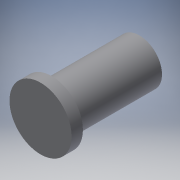
# Autodesk Inventor part: PinLarge
Saved by Autodesk Inventor 2016 (Build 200138000, 138)
## iProperties
Created: 2017-02-20
Part Number: PinLarge
Material: Generic
Document SubType Name: Modeling
Designer: Owner
Density: 1 g/cm^3
Appearance: Default
Author: Owner
Autodesk Inventor part; units mm, degrees
ref_plane "YZ Plane" through (0, 0, 0) normal (1, 0, 0) x (0, 1, 0)
ref_plane "XZ Plane" through (0, 0, 0) normal (0, 1, 0) x (-1, 0, 0)
ref_plane "XY Plane" through (0, 0, 0) normal (0, 0, 1) x (1, 0, 0)
sketch "Sketch1" plane through (0, 0, 0) normal (0, 0, 1) x (1, 0, 0)
  spline S0 degree 3 poles (0, -9.2017) (-0.1549, -9.1123) (-0.2951, -9.003) (-0.5897, -8.7084) (-0.7431, -8.4859) (-0.9483, -7.994) (-1, -7.7245) (-1, -7.2148) (-0.9483, -6.9453) (-0.7431, -6.4535) (-0.5897, -6.2309) (-0.2951, -5.9364) (-0.1549, -5.827) (0, -5.7376) knots 0.101257 0.101257 0.101257 0.101257 0.153157 0.153157 0.229613 0.229613 0.306069 0.306069 0.382525 0.382525 0.458981 0.458981 0.510882 0.510882 0.510882 0.510882 projected
  line L0 (0, -11.8572) -> (0, -9.2017) projected
  line L1 (0, -11.8572) -> (4, -11.8572) projected
  spline S1 degree 3 poles (5, -10.8238) (5, -10.9525) (4.9711, -11.1043) (4.8761, -11.34) (4.7944, -11.4663) (4.6201, -11.6458) (4.4966, -11.7308) (4.2682, -11.8276) (4.1233, -11.8572) (4, -11.8572) knots 0.455708 0.455708 0.455708 0.455708 0.494332 0.494332 0.531937 0.531937 0.569404 0.569404 0.606379 0.606379 0.606379 0.606379 projected
  line L2 (5, -4.1156) -> (5, -10.8238) projected
  spline S2 degree 3 poles (4, -3.0822) (4.1233, -3.0822) (4.2682, -3.1118) (4.4966, -3.2086) (4.6201, -3.2936) (4.7944, -3.4731) (4.8761, -3.5994) (4.9711, -3.8351) (5, -3.9868) (5, -4.1156) knots 0.606379 0.606379 0.606379 0.606379 0.643354 0.643354 0.680821 0.680821 0.718427 0.718427 0.75705 0.75705 0.75705 0.75705 projected
  line L3 (4, -3.0822) -> (0, -3.0822) projected
  line L4 (0, -5.7376) -> (0, -3.0822) projected
  arc A0 (0, -5.7376) -> (0, -9.2017) centre (1, -7.4697) ccw projected
  circle A1 centre (1, -7.4697) radius 2
  point P0 (0, 0)
  dimension "d0" = 4
  constraints: 1 centre point, 1 coincident
  measures "d0" diameter of A1
extrude "Extrusion1" add sketch "Sketch1" along normal blind 7.75 contours S0 A1
sketch "Sketch2" plane through (1, -7.4697, 7.75) normal (0, 0, 1) x (1, 0, 0)
  circle A0 centre (0, 0) radius 2.75
  point P0 (-1, 7.4697)
  dimension "d3" = 5.5
  constraints: 1 centre point
  measures "d3" diameter of A0
extrude "Extrusion2" add sketch "Sketch2" along normal blind 1
body "Solid1"
